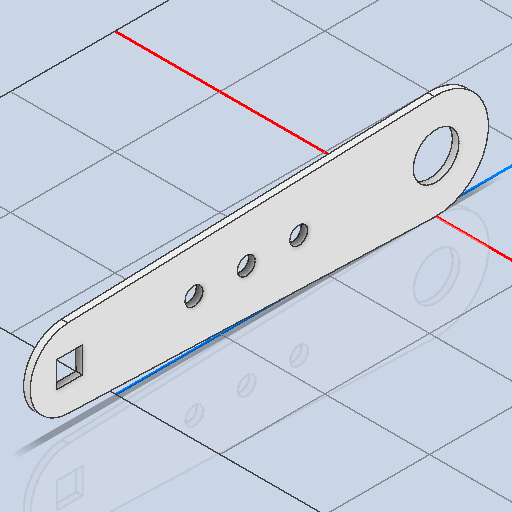
# Autodesk Inventor part: Gusset
Saved by Autodesk Inventor 2026 (Build 300175000, 175)
## iProperties
Created: 2025-04-12
Part Number: Gusset
Material: Acetal Resin, White
Document SubType Name: Modeling
Designer: avere
Density: 1.425 g/cm^3
Appearance: Smooth - White
Author: avere
Autodesk Inventor part; units mm, degrees
ref_plane "YZ Plane" through (0, 0, 0) normal (1, 0, 0) x (0, 1, 0)
ref_plane "XZ Plane" through (0, 0, 0) normal (0, 1, 0) x (-1, 0, 0)
ref_plane "XY Plane" through (0, 0, 0) normal (0, 0, 1) x (1, 0, 0)
sketch "main" plane through (0, 0, 0) normal (0, 0, 1) x (1, 0, 0)
  line L0 (46.0129, -12.1958) -> (-42.8871, -12.1958)
  circle A0 centre (46.0129, -12.1958) radius 5.5563
  arc A1 (45.534, -24.8867) -> (45.5846, 0.497) centre (46.0129, -12.1958) ccw
  line L1 (-46.0418, -15.1681) -> (-39.7426, -15.1681)
  line L2 (-39.7426, -15.1681) -> (-39.7426, -8.8689)
  line L3 (-39.7426, -8.8689) -> (-46.0418, -8.8689)
  line L4 (-46.0418, -8.8689) -> (-46.0418, -15.1681)
  line L5 (-46.0418, -15.1681) -> (-39.7426, -8.8689) construction
  line L6 (-39.7426, -15.1681) -> (-46.0418, -8.8689) construction
  arc A2 (-43.2133, -2.4989) -> (-43.2513, -21.5368) centre (-42.8922, -12.0185) ccw
  line L7 (-43.2133, -2.4989) -> (45.5846, 0.497)
  line L8 (-43.2513, -21.5368) -> (45.534, -24.8867)
  circle A3 centre (12.7, -12.1958) radius 2.1844
  circle A4 centre (0, -12.1958) radius 2.1844
  circle A5 centre (-12.7, -12.1958) radius 2.1844
  point P0 (-14.9546, -14.9924)
  point P1 (-63.2594, -31.7725)
  point P2 (-42.8922, -12.0185)
  dimension "d0" = 88.9
  dimension "d2" = 11.1125
  dimension "d3" = 25.4
  dimension "d4" = 6.2992
  dimension "d5" = 6.2992
  dimension "d6" = 19.05
  dimension "d9" = 4.3688
  dimension "d12" = 12.7
  measures "d0" distance of L0.start L0.end
  measures "d2" diameter of A0
  measures "d3" diameter of A1
  measures "d4" distance of L3.end L2.end
  measures "d5" distance of L2.end L1.end
  measures "d6" diameter of A2
  measures "d9" diameter of A3
  measures "d12" distance of A3.centre A4.centre
sketch "Sketch1" plane through (0, 0, 0) normal (1, 0, 0) x (0, 1, 0)
  line L0 (0, 0) -> (-0.1504, 88.8999)
  circle A0 centre (0, 0) radius 5.5563
  arc A1 (-12.6918, 0.4574) -> (12.692, 0.4497) centre (0, 0) ccw
  line L1 (-3.128, 92.0495) -> (-3.1174, 85.7503)
  line L2 (-3.1174, 85.7503) -> (3.1818, 85.7609)
  line L3 (3.1818, 85.7609) -> (3.1711, 92.0601)
  line L4 (3.1711, 92.0601) -> (-3.128, 92.0495)
  line L5 (-3.128, 92.0495) -> (3.1818, 85.7609) construction
  line L6 (-3.1174, 85.7503) -> (3.1711, 92.0601) construction
  arc A2 (9.5459, 89.2425) -> (-9.4919, 89.2482) centre (0.0269, 88.9052) ccw
  line L7 (9.5459, 89.2425) -> (12.692, 0.4497)
  line L8 (-9.4919, 89.2482) -> (-12.6918, 0.4574)
  circle A3 centre (-0.0563, 33.3128) radius 2.1844
  circle A4 centre (-0.0778, 46.0128) radius 2.1844
  circle A5 centre (-0.0993, 58.7128) radius 2.1844
  point P0 (0, 0)
  constraints: 1 other
extrude "Extrusion1" add sketch "Sketch1" along normal blind 1.5875
body "Solid1"
